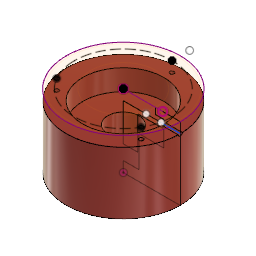
CNC Switched tool Setter v4 (Autodesk Fusion 360 design; units mm, degrees)
Autodesk Fusion 360 part; units mm, degrees
sketch "Sketch1" plane through (0, 0, 0) normal (0, 1, 0) x (1, 0, 0)
  line L0 (0, 0) -> (27.5, 0)
  line L1 (27.5, 0) -> (27.5, -30)
  line L2 (27.5, -30) -> (19.5, -30)
  line L3 (19.5, -30) -> (19.5, -20)
  line L4 (19.5, -20) -> (7.5, -20)
  line L5 (7.5, -20) -> (7.5, -5)
  line L6 (7.5, -5) -> (0, -5)
  line L7 (0, -5) -> (0, 0)
  line L8 (19, -30) -> (19, -28)
  line L9 (19, -28) -> (7, -28)
  line L10 (7, -28) -> (7, -12)
  line L11 (7, -12) -> (0, -12)
  line L12 (0, -12) -> (0, -30)
  line L13 (0, -30) -> (19, -30)
  line L14 (27.5, -30) -> (18.2223, -30)
  line L15 (27.5, -35) -> (27.5, -30)
  line L16 (15.5, -35) -> (15.5, -32)
  line L17 (11, -30) -> (27.5, -30)
  line L18 (15.5, -35) -> (27.5, -35)
  line L19 (19.5, -30) -> (19.5, -32)
  line L20 (19.5, -32) -> (15.5, -32)
  dimension "d1" = 7.5
  dimension "d2" = 27.5
  dimension "d3" = 30
  dimension "d4" = 8
  dimension "d5" = 10
  dimension "d6" = 5
  dimension "d8" = 19
  dimension "d9" = 2
  dimension "d10" = 18
  dimension "d11" = 7
  dimension "d13" = 12
  dimension "d15" = 3
  dimension "d16" = 2
  dimension "d21" = 11
  measures "d1" distance of L5 L7
  measures "d2" distance of L1 L7
  measures "d4" distance of L0.start
  measures "d6" distance of L0.start
  measures "d8" distance of L8 L12
  measures "d10" distance of L0.start
  measures "d13" distance of L0.start
  measures "d21" distance of L7 L16
revolve "Revolve1" add sketch "Sketch1" angle 360 about axis through (0, 0, 1.75) along (0, 0, 1) contours L0 L1 L2 L3 L4 L5 L6 L7 L14 L17 makes body 1
revolve "Revolve2" add sketch "Sketch1" angle 360 about axis through (0, 0, 5) along (0, 0, -1) separate body contours L2 L14 L15 L16 L17 L18 L19 L20 makes body 2
revolve "Revolve3" add sketch "Sketch1" angle 360 about axis through (0, 0, 12) along (0, 0, 1) separate body contours L8 L9 L10 L11 L12 L13 L14 L17 makes body 3
chamfer "Chamfer1" distance 2 angle 45 1 edges at (-6.5263, -2.5313, 12) on bodies 3
chamfer "Chamfer2" distance 1 angle 45 1 edges at (-25.639, -9.9444, 35) on bodies 2
sketch "Sketch2" plane through (0, 0, 35) normal (0, 0, 1) x (-1, 0, 0)
  circle A0 centre (0, 0) radius 15.5
  circle A1 centre (0, 0) radius 26.5
  circle A2 centre (0, 0) radius 23.5 construction
  circle A3 centre (0, 0) radius 27.5
  line L0 (0, 0) -> (-19, 0)
  line L1 (0, 0) -> (0, -32) construction
  circle A4 centre (0, -23.5) radius 1
  circle A5 centre (20.3516, 11.75) radius 1
  circle A6 centre (-20.3516, 11.75) radius 1
  dimension "d22" = 2
  dimension "d24" = 360
  dimension "d30" = 50
  dimension "d31" = 32
  dimension "d32" = 47
  measures "d22" diameter of A4
  measures "d32" diameter of A2
hole "Hole1" at (-20.3516, -11.75, 35) at (0, 23.5, 35) at (20.3516, -11.75, 35) direction (0, 0, -1) diameter 2 depth 16 tip angle 118 countersink diameter 6 countersink angle 90 bodies 1 2 3
hole "Hole2" at (27.5, 0, 29.9966) direction (-1, 0, 0) diameter 2 depth 10 tip angle 118 bodies 1 2
component "Body" placed x (1, 0, 0) y (0, 1, 0) z (0, 0, 1) at (0, 0, 0)
component "Retaininer" placed x (1, 0, 0) y (0, 1, 0) z (0, 0, 1) at (0, 0, 0)
component "Plunger" placed x (1, 0, 0) y (0, 1, 0) z (0, 0, 1) at (0, 0, 0)
hidden bodies 2 3
equation "d1 = ( 15 / 2 ) * 1 mm"
equation "d2 = ( 55 / 2 ) * 1 mm"
equation "d8 = d2 - d4 - 0.5 mm"
equation "d10 = d3 - d5 - 2 mm"
equation "d11 = d1 - 0.5 mm"
equation "d13 = d4 + 4 mm"
equation "d32 = 55 mm - 8 mm"
